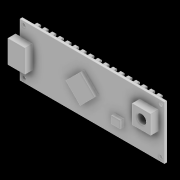
# Autodesk Inventor part: arduino
Saved by Autodesk Inventor 2020 (Build 240168000, 168)
## iProperties
Created: 2020-01-13
Part Number: arduino
Material: Generic
Document SubType Name: Modeling
Designer: valer
Density: 1 g/cm^3
Appearance: Default
Author: valer
Autodesk Inventor part; units mm, degrees
ref_plane "YZ Plane" through (0, 0, 0) normal (1, 0, 0) x (0, 1, 0)
ref_plane "XZ Plane" through (0, 0, 0) normal (0, 1, 0) x (-1, 0, 0)
ref_plane "XY Plane" through (0, 0, 0) normal (0, 0, 1) x (1, 0, 0)
sketch "TopProfile" plane through (0, 0, 0) normal (0, 0, 1) x (1, 0, 0)
  line L0 (0, 0) -> (48.26, 0)
  line L1 (48.26, 0) -> (48.26, 17.78)
  line L2 (48.26, 17.78) -> (0, 17.78)
  line L3 (0, 17.78) -> (0, 0)
  circle A0 centre (1.27, 16.51) radius 1.27
  circle A1 centre (46.99, 16.51) radius 1.27
  circle A2 centre (1.27, 1.27) radius 1.27
  circle A3 centre (46.99, 1.27) radius 1.27
  line L4 (16.5608, 8.8667) -> (21.4101, 13.716)
  line L5 (21.4101, 13.716) -> (26.2595, 8.8667)
  line L6 (26.2595, 8.8667) -> (21.4101, 4.0173)
  line L7 (21.4101, 4.0173) -> (16.5608, 8.8667)
  line L8 (40.005, 14.6304) -> (46.228, 14.6304)
  line L9 (46.228, 14.6304) -> (46.228, 8.4074)
  line L10 (46.228, 8.4074) -> (40.005, 8.4074)
  line L11 (40.005, 8.4074) -> (40.005, 14.6304)
  line L12 (43.1165, 14.6304) -> (43.1165, 8.4074) construction
  line L13 (40.005, 11.5189) -> (46.228, 11.5189) construction
  circle A4 centre (43.1165, 11.5189) radius 1.5875
  line L14 (4.2273, 12.7) -> (-1.4877, 12.7)
  line L15 (-1.4877, 12.7) -> (-1.4877, 5.08)
  line L16 (-1.4877, 5.08) -> (4.2273, 5.08)
  line L17 (4.2273, 5.08) -> (4.2273, 12.7)
  line L18 (-1.4877, 8.89) -> (4.2273, 8.89) construction
  line L19 (31.75, 6.35) -> (34.798, 6.35)
  line L20 (34.798, 6.35) -> (34.798, 3.9298)
  line L21 (34.798, 3.9298) -> (31.75, 3.9298)
  line L22 (31.75, 3.9298) -> (31.75, 6.35)
  line L23 (3.175, 16.9342) -> (4.445, 16.9342)
  line L24 (4.445, 16.9342) -> (4.445, 16.4262)
  line L25 (4.445, 16.4262) -> (3.175, 16.4262)
  line L26 (3.175, 16.4262) -> (3.175, 16.9342)
  line L27 (5.715, 16.4262) -> (5.715, 16.9342)
  line L28 (5.715, 16.9342) -> (6.985, 16.9342)
  line L29 (6.985, 16.4262) -> (5.715, 16.4262)
  line L30 (6.985, 16.9342) -> (6.985, 16.4262)
  line L31 (8.255, 16.4262) -> (8.255, 16.9342)
  line L32 (8.255, 16.9342) -> (9.525, 16.9342)
  line L33 (9.525, 16.4262) -> (8.255, 16.4262)
  line L34 (9.525, 16.9342) -> (9.525, 16.4262)
  line L35 (10.795, 16.4262) -> (10.795, 16.9342)
  line L36 (10.795, 16.9342) -> (12.065, 16.9342)
  line L37 (12.065, 16.4262) -> (10.795, 16.4262)
  line L38 (12.065, 16.9342) -> (12.065, 16.4262)
  line L39 (13.335, 16.4262) -> (13.335, 16.9342)
  line L40 (13.335, 16.9342) -> (14.605, 16.9342)
  line L41 (14.605, 16.4262) -> (13.335, 16.4262)
  line L42 (14.605, 16.9342) -> (14.605, 16.4262)
  line L43 (15.875, 16.4262) -> (15.875, 16.9342)
  line L44 (15.875, 16.9342) -> (17.145, 16.9342)
  line L45 (17.145, 16.4262) -> (15.875, 16.4262)
  line L46 (17.145, 16.9342) -> (17.145, 16.4262)
  line L47 (18.415, 16.4262) -> (18.415, 16.9342)
  line L48 (18.415, 16.9342) -> (19.685, 16.9342)
  line L49 (19.685, 16.4262) -> (18.415, 16.4262)
  line L50 (19.685, 16.9342) -> (19.685, 16.4262)
  line L51 (20.955, 16.4262) -> (20.955, 16.9342)
  line L52 (20.955, 16.9342) -> (22.225, 16.9342)
  line L53 (22.225, 16.4262) -> (20.955, 16.4262)
  line L54 (22.225, 16.9342) -> (22.225, 16.4262)
  line L55 (23.495, 16.4262) -> (23.495, 16.9342)
  line L56 (23.495, 16.9342) -> (24.765, 16.9342)
  line L57 (24.765, 16.4262) -> (23.495, 16.4262)
  line L58 (24.765, 16.9342) -> (24.765, 16.4262)
  line L59 (26.035, 16.4262) -> (26.035, 16.9342)
  line L60 (26.035, 16.9342) -> (27.305, 16.9342)
  line L61 (27.305, 16.4262) -> (26.035, 16.4262)
  line L62 (27.305, 16.9342) -> (27.305, 16.4262)
  line L63 (28.575, 16.4262) -> (28.575, 16.9342)
  line L64 (28.575, 16.9342) -> (29.845, 16.9342)
  line L65 (29.845, 16.4262) -> (28.575, 16.4262)
  line L66 (29.845, 16.9342) -> (29.845, 16.4262)
  line L67 (31.115, 16.4262) -> (31.115, 16.9342)
  line L68 (31.115, 16.9342) -> (32.385, 16.9342)
  line L69 (32.385, 16.4262) -> (31.115, 16.4262)
  line L70 (32.385, 16.9342) -> (32.385, 16.4262)
  line L71 (33.655, 16.4262) -> (33.655, 16.9342)
  line L72 (33.655, 16.9342) -> (34.925, 16.9342)
  line L73 (34.925, 16.4262) -> (33.655, 16.4262)
  line L74 (34.925, 16.9342) -> (34.925, 16.4262)
  line L75 (36.195, 16.4262) -> (36.195, 16.9342)
  line L76 (36.195, 16.9342) -> (37.465, 16.9342)
  line L77 (37.465, 16.4262) -> (36.195, 16.4262)
  line L78 (37.465, 16.9342) -> (37.465, 16.4262)
  line L79 (38.735, 16.4262) -> (38.735, 16.9342)
  line L80 (38.735, 16.9342) -> (40.005, 16.9342)
  line L81 (40.005, 16.4262) -> (38.735, 16.4262)
  line L82 (40.005, 16.9342) -> (40.005, 16.4262)
  line L83 (41.275, 16.4262) -> (41.275, 16.9342)
  line L84 (41.275, 16.9342) -> (42.545, 16.9342)
  line L85 (42.545, 16.4262) -> (41.275, 16.4262)
  line L86 (42.545, 16.9342) -> (42.545, 16.4262)
  line L87 (43.815, 16.4262) -> (43.815, 16.9342)
  line L88 (43.815, 16.9342) -> (45.085, 16.9342)
  line L89 (45.085, 16.4262) -> (43.815, 16.4262)
  line L90 (45.085, 16.9342) -> (45.085, 16.4262)
  line L91 (3.175, 0.8458) -> (4.445, 0.8458)
  line L92 (4.445, 0.8458) -> (4.445, 1.3538)
  line L93 (4.445, 1.3538) -> (3.175, 1.3538)
  line L94 (3.175, 1.3538) -> (3.175, 0.8458)
  line L95 (5.715, 1.3538) -> (5.715, 0.8458)
  line L96 (5.715, 0.8458) -> (6.985, 0.8458)
  line L97 (6.985, 1.3538) -> (5.715, 1.3538)
  line L98 (6.985, 0.8458) -> (6.985, 1.3538)
  line L99 (8.255, 1.3538) -> (8.255, 0.8458)
  line L100 (8.255, 0.8458) -> (9.525, 0.8458)
  line L101 (9.525, 1.3538) -> (8.255, 1.3538)
  line L102 (9.525, 0.8458) -> (9.525, 1.3538)
  line L103 (10.795, 1.3538) -> (10.795, 0.8458)
  line L104 (10.795, 0.8458) -> (12.065, 0.8458)
  line L105 (12.065, 1.3538) -> (10.795, 1.3538)
  line L106 (12.065, 0.8458) -> (12.065, 1.3538)
  line L107 (13.335, 1.3538) -> (13.335, 0.8458)
  line L108 (13.335, 0.8458) -> (14.605, 0.8458)
  line L109 (14.605, 1.3538) -> (13.335, 1.3538)
  line L110 (14.605, 0.8458) -> (14.605, 1.3538)
  line L111 (15.875, 1.3538) -> (15.875, 0.8458)
  line L112 (15.875, 0.8458) -> (17.145, 0.8458)
  line L113 (17.145, 1.3538) -> (15.875, 1.3538)
  line L114 (17.145, 0.8458) -> (17.145, 1.3538)
  line L115 (18.415, 1.3538) -> (18.415, 0.8458)
  line L116 (18.415, 0.8458) -> (19.685, 0.8458)
  line L117 (19.685, 1.3538) -> (18.415, 1.3538)
  line L118 (19.685, 0.8458) -> (19.685, 1.3538)
  line L119 (20.955, 1.3538) -> (20.955, 0.8458)
  line L120 (20.955, 0.8458) -> (22.225, 0.8458)
  line L121 (22.225, 1.3538) -> (20.955, 1.3538)
  line L122 (22.225, 0.8458) -> (22.225, 1.3538)
  line L123 (23.495, 1.3538) -> (23.495, 0.8458)
  line L124 (23.495, 0.8458) -> (24.765, 0.8458)
  line L125 (24.765, 1.3538) -> (23.495, 1.3538)
  line L126 (24.765, 0.8458) -> (24.765, 1.3538)
  line L127 (26.035, 1.3538) -> (26.035, 0.8458)
  line L128 (26.035, 0.8458) -> (27.305, 0.8458)
  line L129 (27.305, 1.3538) -> (26.035, 1.3538)
  line L130 (27.305, 0.8458) -> (27.305, 1.3538)
  line L131 (28.575, 1.3538) -> (28.575, 0.8458)
  line L132 (28.575, 0.8458) -> (29.845, 0.8458)
  line L133 (29.845, 1.3538) -> (28.575, 1.3538)
  line L134 (29.845, 0.8458) -> (29.845, 1.3538)
  line L135 (31.115, 1.3538) -> (31.115, 0.8458)
  line L136 (31.115, 0.8458) -> (32.385, 0.8458)
  line L137 (32.385, 1.3538) -> (31.115, 1.3538)
  line L138 (32.385, 0.8458) -> (32.385, 1.3538)
  line L139 (33.655, 1.3538) -> (33.655, 0.8458)
  line L140 (33.655, 0.8458) -> (34.925, 0.8458)
  line L141 (34.925, 1.3538) -> (33.655, 1.3538)
  line L142 (34.925, 0.8458) -> (34.925, 1.3538)
  line L143 (36.195, 1.3538) -> (36.195, 0.8458)
  line L144 (36.195, 0.8458) -> (37.465, 0.8458)
  line L145 (37.465, 1.3538) -> (36.195, 1.3538)
  line L146 (37.465, 0.8458) -> (37.465, 1.3538)
  line L147 (38.735, 1.3538) -> (38.735, 0.8458)
  line L148 (38.735, 0.8458) -> (40.005, 0.8458)
  line L149 (40.005, 1.3538) -> (38.735, 1.3538)
  line L150 (40.005, 0.8458) -> (40.005, 1.3538)
  line L151 (41.275, 1.3538) -> (41.275, 0.8458)
  line L152 (41.275, 0.8458) -> (42.545, 0.8458)
  line L153 (42.545, 1.3538) -> (41.275, 1.3538)
  line L154 (42.545, 0.8458) -> (42.545, 1.3538)
  line L155 (43.815, 1.3538) -> (43.815, 0.8458)
  line L156 (43.815, 0.8458) -> (45.085, 0.8458)
  line L157 (45.085, 1.3538) -> (43.815, 1.3538)
  line L158 (45.085, 0.8458) -> (45.085, 1.3538)
  circle A5 centre (1.27, 16.51) radius 0.635
  circle A6 centre (1.27, 1.27) radius 0.635
  circle A7 centre (46.99, 16.51) radius 0.635
  circle A8 centre (46.99, 1.27) radius 0.635
  point P0 (0, 8.89)
  dimension "d0" = 48.26
  dimension "d1" = 17.78
  dimension "d2" = 2.54
  dimension "d3" = 6.858
  dimension "d4" = 45
  dimension "d5" = 4.064
  dimension "d6" = 6.223
  dimension "d7" = 3.1496
  dimension "d8" = 2.032
  dimension "d9" = 3.175
  dimension "d10" = 5.715
  dimension "d11" = 7.62
  dimension "d12" = 1.4877
  dimension "d13" = 16.5608
  dimension "d14" = 3.048
  dimension "d15" = 2.4202
  dimension "d16" = 11.43
  dimension "d17" = 13.462
  dimension "d18" = 0.508
  dimension "d19" = 1.27
  dimension "d20" = 3.175
  dimension "d21" = 0.8458
  dimension "d24" = 2.54
  dimension "d29" = 1.27
  constraints: 318 end point, 68 symmetric about line, 12 parallel, 9 centre point, 8 midpoint, 8 perpendicular, 8 tangent, 6 equal radius, 6 horizontal, 4 coincident, 1 point on line, 128 other
  measures "d0" distance of L1.end L2.end
  measures "d1" distance of L2.end L0.start
  measures "d2" diameter of A0
  measures "d3" distance of L4.end L5.end
  measures "d4" angle of L2 L4
  measures "d5" distance from line of L2 L4.end
  measures "d6" distance of L8.end L9.end
  measures "d7" distance between parallel lines of L2 L8
  measures "d8" distance between parallel lines of L1 L9
  measures "d9" diameter of A4
  measures "d10" distance of L14.start L14.end
  measures "d11" distance of L16.end L14.start
  measures "d12" distance between parallel lines of L15 L3
  measures "d13" distance from line of L3 L4.start
  measures "d14" distance of L19.start L19.end
  measures "d15" distance of L21.end L19.start
  measures "d16" distance between parallel lines of L2 L19
  measures "d17" distance between parallel lines of L1 L20
  measures "d18" distance of L23.end L24.end
  measures "d19" distance of L23.start L23.end
  measures "d20" distance between parallel lines of L3 L26
  measures "d21" distance between parallel lines of L2 L23
  measures "d24" distance of L25.end L27.start
  measures "d29" diameter of A5
extrude "BaseFeature" add sketch "TopProfile" against normal blind 0.7937 contours L3 A2 L0 | A2 L3 L16 L17 L14 A0 L2 A1 L1 A3 L0 | A2 | A3 L1 L0 | A3 | L3 L14 L17 L16 | A1 L2 L1 | A1 | L3 L2 A0 | A0 | L4 L5 L6 L7 | L8 L9 L10 L11 | A4 | L19 L20 L21 L22 | L23 L24 L25 L26 | L27 L28 L30 L29 | L31 L32 L34 L33 | L35 L36 L38 L37 | L39 L40 L42 L41 | L43 L44 L46 L45 | L47 L48 L50 L49 | L51 L52 L54 L53 | L55 L56 L58 L57 | L59 L60 L62 L61 | L63 L64 L66 L65 | L67 L68 L70 L69 | L71 L72 L74 L73 | L75 L76 L78 L77 | L79 L80 L82 L81 | L83 L84 L86 L85 | L87 L88 L90 L89 | L94 L93 L92 L91 | L97 L98 L96 L95 | L101 L102 L100 L99 | L105 L106 L104 L103 | L109 L110 L108 L107 | L113 L114 L112 L111 | L117 L118 L116 L115 | L121 L122 L120 L119 | L125 L126 L124 L123 | L129 L130 L128 L127 | L133 L134 L132 L131 | L137 L138 L136 L135 | L141 L142 L140 L139 | L145 L146 L144 L143 | L149 L150 L148 L147 | L153 L154 L152 L151 | L157 L158 L156 L155 | A5 | A6 | A7 | A8
extrude "UsbFeature" add sketch "TopProfile" along normal blind 2.54 contours L16 L15 L14 L3 | L3 L14 L17 L16 | L8 L9 L10 L11
extrude "ChipsFeature" add sketch "TopProfile" along normal blind 1.27 contours L4 L5 L6 L7 | L19 L20 L21 L22
hole "MountHolesFeature" at (1.27, 16.51, 0) at (1.27, 1.27, 0) at (46.99, 16.51, 0) at (46.99, 1.27, 0) direction (0, 0, -1) diameter 1.27 end through all
extrude "Extrusion4" add sketch "TopProfile" against normal blind 2.54 contours L23 L24 L25 L26 | L27 L28 L30 L29 | L31 L32 L34 L33 | L35 L36 L38 L37 | L39 L40 L42 L41 | L43 L44 L46 L45 | L47 L48 L50 L49 | L51 L52 L54 L53 | L55 L56 L58 L57 | L59 L60 L62 L61 | L63 L64 L66 L65 | L67 L68 L70 L69 | L71 L72 L74 L73 | L75 L76 L78 L77 | L79 L80 L82 L81 | L83 L84 L86 L85 | L87 L88 L90 L89 | L94 L93 L92 L91 | L97 L98 L96 L95 | L101 L102 L100 L99 | L105 L106 L104 L103 | L109 L110 L108 L107 | L113 L114 L112 L111 | L117 L118 L116 L115 | L121 L122 L120 L119 | L125 L126 L124 L123 | L129 L130 L128 L127 | L133 L134 L132 L131 | L137 L138 L136 L135 | L141 L142 L140 L139 | L145 L146 L144 L143 | L149 L150 L148 L147 | L153 L154 L152 L151 | L157 L158 L156 L155
body "Solid1"
